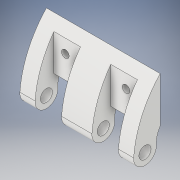
# Autodesk Inventor part: TC006b
Saved by Autodesk Inventor 2017 SP1 (Build 210196100, 196)
## iProperties
Created: 2018-01-07
Part Number: TC006b
Material: ABS Plastic
Document SubType Name: Modeling
Designer: Zach
Density: 1.06 g/cm^3
Appearance: CR White
Author: Zach
Autodesk Inventor part; units mm, degrees
ref_plane "YZ Plane" through (0, 0, 0) normal (1, 0, 0) x (0, 1, 0)
ref_plane "XZ Plane" through (0, 0, 0) normal (0, 1, 0) x (-1, 0, 0)
ref_plane "XY Plane" through (0, 0, 0) normal (0, 0, 1) x (1, 0, 0)
sketch "Sketch1" plane through (0, 0, 0) normal (0, 0, 1) x (1, 0, 0)
  line L0 (0, 0) -> (75, 0)
  line L1 (75, 0) -> (75, 30)
  line L2 (75, 30) -> (0, 30)
  line L3 (0, 30) -> (0, 0)
  circle A0 centre (17.5, 15) radius 2.5
  circle A1 centre (57.5, 15) radius 2.5
  line L4 (17.5, 15) -> (57.5, 15) construction
  point P0 (37.5, 15)
  point P1 (37.5, 30)
  dimension "d0" = 75
  dimension "d1" = 30
  dimension "d2" = 5
  dimension "d3" = 5
  dimension "d4" = 40
  dimension "d5" = 15
  constraints: 10 end point, 2 centre point, 2 horizontal, 2 midpoint, 2 parallel, 1 perpendicular, 1 vertical alignment
  measures "d0" distance of L2.end L1.end
  measures "d1" distance of L1.end L0.end
  measures "d2" diameter of A0
  measures "d3" diameter of A1
  measures "d4" distance of L4.end L4.start
  measures "d5" distance between parallel lines of L0 L4
extrude "Extrusion1" add sketch "Sketch1" along normal blind 5
sketch "Sketch2" plane through (75, 0, 0) normal (1, 0, 0) x (0, 0, -1)
  circle A0 centre (-15, -10) radius 4
  circle A1 centre (-15, -10) radius 7.5 construction
  line L0 (-5, 0) -> (-5, 30) construction
  arc A2 (-5, 30) -> (-22.4763, -9.4047) centre (42.3186, -14.564) ccw
  arc A3 (-5, 0) -> (-7.5195, -9.4597) centre (7.4415, -8.379) ccw
  arc A4 (-22.4763, -9.4047) -> (-7.5195, -9.4597) centre (-15, -10) ccw
  line L1 (0, 0) -> (-5, 0) projected
  line L2 (0, 30) -> (-5, 30) projected
  line L3 (-5, 30) -> (-5, 0)
  dimension "d8" = 8
  dimension "d9" = 15
  dimension "d10" = 10
  dimension "d11" = 10
  dimension "d12" = 65
  dimension "d13" = 15
  constraints: 8 point on circle, 5 centre point, 4 tangent, 2 end point, 1 coincident, 1 perpendicular
  measures "d8" diameter of A0
  measures "d9" diameter of A1
  measures "d10" distance from line of L1 A0.centre
  measures "d11" distance from line of L0 A0.centre
  measures "d12" radius of A2
  measures "d13" radius of A3
extrude "Extrusion2" add sketch "Sketch2" against normal blind 10
sketch "Sketch3" plane through (0, 0, 0) normal (-1, 0, 0) x (0, 0, 1)
  circle A0 centre (15, -10) radius 4 projected
  arc A1 (7.5195, -9.4597) -> (5, 0) centre (-7.4415, -8.379) ccw projected
  arc A2 (7.5195, -9.4597) -> (22.4763, -9.4047) centre (15, -10) ccw projected
  arc A3 (22.4763, -9.4047) -> (5, 30) centre (-42.3186, -14.564) ccw projected
  line L0 (5, 0) -> (5, 30) projected
  point P0 (0, 0)
extrude "Extrusion3" add sketch "Sketch3" against normal blind 10
ref_plane "Work Plane1" through (37.5, 0, 0) normal (-1, 0, 0) x (0, 0, 1)
sketch "Sketch4" plane through (37.5, 0, 0) normal (-1, 0, 0) x (0, 0, 1)
  circle A0 centre (15, -10) radius 4 projected
  arc A1 (7.5195, -9.4597) -> (5, 0) centre (-7.4415, -8.379) ccw projected
  arc A2 (7.5195, -9.4597) -> (22.4763, -9.4047) centre (15, -10) ccw projected
  arc A3 (22.4763, -9.4047) -> (5, 30) centre (-42.3186, -14.564) ccw projected
  line L0 (5, 0) -> (5, 30) projected
  point P0 (0, 0)
extrude "Extrusion4" add sketch "Sketch4" along normal mid plane 20
sketch "Sketch5" plane through (0, 0, 5) normal (0, 0, 1) x (1, 0, 0)
  circle A0 centre (17.5, 15) radius 2.5 projected
  line L0 (27.5, 0) -> (27.5, 30) projected
  line L1 (27.5, 30) -> (10, 30) projected
  line L2 (10, 30) -> (10, 0) projected
  line L3 (10, 0) -> (27.5, 0) projected
  line L4 (47.5, 30) -> (47.5, 0) projected
  line L5 (47.5, 0) -> (65, 0) projected
  line L6 (65, 0) -> (65, 30) projected
  line L7 (65, 30) -> (47.5, 30) projected
  circle A1 centre (57.5, 15) radius 2.5 projected
  point P0 (0, 0)
extrude "Extrusion5" add sketch "Sketch5" along normal blind 5
sketch "Sketch6" plane through (75, 0, 0) normal (1, 0, 0) x (0, 0, -1)
  line L0 (0, 0) -> (-5, 0) projected
  line L1 (0, 30) -> (-5, 30) projected
  line L2 (0, 0) -> (-5, 0)
  line L3 (-5, 0) -> (-5, 30)
  line L4 (-5, 30) -> (0, 30)
  line L5 (0, 30) -> (0, 0)
  arc A0 (-5, 30) -> (-10, 24.0076) centre (42.3186, -14.564) ccw projected
  line L6 (-5, 30) -> (-10, 30) projected
  line L7 (-10, 24.0076) -> (-10, 30) projected
  constraints: 8 end point, 2 parallel, 1 horizontal, 1 perpendicular
extrude "Extrusion6" cut sketch "Sketch6" against normal through all
body "Solid1"
